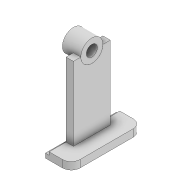
# Autodesk Inventor part: lllll
Saved by Autodesk Inventor 2021 (Build 250183000, 183)
## iProperties
Created: 2021-06-28
Part Number: lllll
Material: Generic
Document SubType Name: Modeling
Designer: Shaheen Khan
Density: 1 g/cm^3
Appearance: Default
Author: Shaheen Khan
Autodesk Inventor part; units mm, degrees
ref_plane "YZ Plane" through (0, 0, 0) normal (1, 0, 0) x (0, 1, 0)
ref_plane "XZ Plane" through (0, 0, 0) normal (0, 1, 0) x (-1, 0, 0)
ref_plane "XY Plane" through (0, 0, 0) normal (0, 0, 1) x (1, 0, 0)
sketch "Sketch1" plane through (0, 0, 0) normal (0, 1, 0) x (-1, 0, 0)
  line L0 (-17.5, 48) -> (17.5, 48)
  line L1 (17.5, 48) -> (17.5, -48)
  line L2 (17.5, -48) -> (-17.5, -48)
  line L3 (-17.5, -48) -> (-17.5, 48)
  line L4 (-17.5, 48) -> (17.5, -48) construction
  line L5 (17.5, 48) -> (-17.5, -48) construction
  point P0 (0, 0)
  dimension "d0" = 96
  dimension "d1" = 35
  constraints: 12 end point, 2 midpoint, 2 parallel, 1 horizontal, 1 perpendicular
  measures "d0" distance of L0.end L1.end
  measures "d1" distance of L0.start L0.end
extrude "Extrusion1" add sketch "Sketch1" along normal blind 10
fillet "Fillet1" radius 12 2 edges at (17.5, 5, -48) (17.5, 5, 48)
sketch "Sketch2" plane through (-17.5, 0, -48) normal (0, 0, -1) x (-1, 0, 0)
  line L0 (0, 0) -> (0, 10) projected
  line L1 (0, 10) -> (-5, 10)
  line L2 (-5, 10) -> (-5, 6)
  line L3 (-5, 6) -> (0, 6)
  line L4 (0, 6) -> (0, 10)
  line L5 (-23, 0) -> (0, 0) projected
  point P0 (-17.5, 0)
  point P1 (0, 6)
  dimension "d5" = 6
  dimension "d6" = 5
  constraints: 8 end point, 2 parallel, 1 horizontal, 1 perpendicular
  measures "d5" distance between parallel lines of L5 L3
  measures "d6" distance from line of L3.end L2
extrude "Extrusion2" cut sketch "Sketch2" against normal through all
sketch "Sketch3" plane through (0, 0, 0) normal (0, 0, 1) x (1, 0, 0)
  line L0 (-12.5, 10) -> (-2.5, 10)
  line L1 (-2.5, 10) -> (-2.5, 110)
  line L2 (-2.5, 110) -> (-12.5, 110)
  line L3 (-12.5, 110) -> (-12.5, 10)
  point P0 (0, 0)
  dimension "d9" = 10
  dimension "d10" = 100
  constraints: 8 end point, 2 parallel, 1 horizontal, 1 perpendicular
  measures "d9" distance of L2.end L1.end
  measures "d10" distance of L0.end L1.end
extrude "Extrusion3" add sketch "Sketch3" along normal mid plane 50
sketch "Sketch4" plane through (-2.5, 10, 25) normal (1, 0, 0) x (0, 0, -1)
  line L0 (50, 100) -> (0, 100) projected
  arc A0 (10, 100) -> (40, 100) centre (25, 100) ccw
  point P0 (25, -10)
  dimension "d13" = 30
  constraints: 2 point on circle, 2 point on line, 1 centre point, 1 midpoint
  measures "d13" diameter of A0
extrude "Extrusion4" cut sketch "Sketch4" against normal blind 50
sketch "Sketch5" plane through (-2.5, 10, 25) normal (1, 0, 0) x (0, 0, -1)
  arc A0 (10, 100) -> (40, 100) centre (25, 100) ccw projected
  circle A1 centre (25, 100) radius 15
  circle A2 centre (25, 100) radius 7.5
  point P0 (25, -10)
  dimension "d16" = 30
  dimension "d17" = 15
  constraints: 2 centre point, 2 coincident
  measures "d16" diameter of A1
  measures "d17" diameter of A2
extrude "Extrusion5" add sketch "Sketch5" against normal blind 25 separate body
body "Solid1"
body "Solid2"
